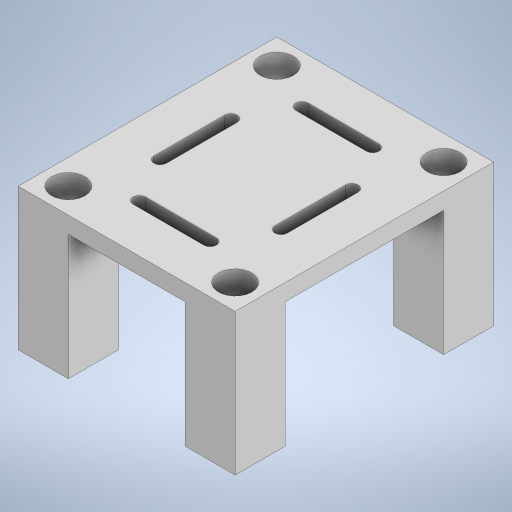
# Autodesk Inventor part: wires_keeper
Saved by Autodesk Inventor 2023 (Build 270158000, 158)
## iProperties
Created: 2023-11-26
Part Number: wires_keeper
Material: Ogólny
Document SubType Name: Modeling
Designer: janek
Density: 1 g/cm^3
Appearance: Domyślna
Author: janek
## iProperties of the stored document wires_keeper_Drukowanie 3D.ipt
Created: 2023-11-26
Part Number: wires_keeper_Drukowanie 3D
Material: Ogólny
Document SubType Name: Modeling
Designer: janek
Density: 1 g/cm^3
Appearance: Domyślna
Author: janek
Autodesk Inventor part; units mm, degrees
ref_plane "YZ Plane" through (0, 0, 0) normal (1, 0, 0) x (0, 1, 0)
ref_plane "XZ Plane" through (0, 0, 0) normal (0, 1, 0) x (-1, 0, 0)
ref_plane "XY Plane" through (0, 0, 0) normal (0, 0, 1) x (1, 0, 0)
sketch "Szkic1" plane through (0, 0, 0) normal (0, 1, 0) x (-1, 0, 0)
  line L0 (20, 25) -> (-20, 25)
  line L1 (-20, 25) -> (-20, -25)
  line L2 (-20, -25) -> (20, -25)
  line L3 (20, -25) -> (20, 25)
  line L4 (20, 25) -> (-20, -25) construction
  line L5 (-20, 25) -> (20, -25) construction
  line L6 (26, 31) -> (14, 31)
  line L7 (14, 31) -> (14, 19)
  line L8 (14, 19) -> (26, 19)
  line L9 (26, 19) -> (26, 31)
  line L10 (26, 31) -> (14, 19) construction
  line L11 (14, 31) -> (26, 19) construction
  line L12 (26, -19) -> (14, -19)
  line L13 (14, -19) -> (14, -31)
  line L14 (14, -31) -> (26, -31)
  line L15 (26, -31) -> (26, -19)
  line L16 (26, -19) -> (14, -31) construction
  line L17 (14, -19) -> (26, -31) construction
  line L18 (-14, 31) -> (-26, 31)
  line L19 (-26, 31) -> (-26, 19)
  line L20 (-26, 19) -> (-14, 19)
  line L21 (-14, 19) -> (-14, 31)
  line L22 (-14, 31) -> (-26, 19) construction
  line L23 (-26, 31) -> (-14, 19) construction
  line L24 (-14, -19) -> (-26, -19)
  line L25 (-26, -19) -> (-26, -31)
  line L26 (-26, -31) -> (-14, -31)
  line L27 (-14, -31) -> (-14, -19)
  line L28 (-14, -19) -> (-26, -31) construction
  line L29 (-26, -19) -> (-14, -31) construction
  point P0 (0, 0)
  point P1 (20, 19)
  point P2 (-14, -25)
  point P3 (-26, -25)
  point P4 (-20, -19)
  point P5 (-20, -31)
  dimension "d0" = 50
  dimension "d1" = 40
  dimension "d2" = 12
  dimension "d3" = 12
  dimension "d4" = 12
  dimension "d5" = 12
  dimension "d6" = 12
  dimension "d7" = 12
  dimension "d8" = 12
  dimension "d9" = 12
  constraints: 60 end point, 15 midpoint, 10 parallel, 5 horizontal, 5 perpendicular
  measures "d0" distance between parallel lines of L0 L2
  measures "d1" distance between parallel lines of L3 L1
  measures "d2" distance of L8.end L7.end
  measures "d3" distance from line of point (20, 19) L6
  measures "d4" distance of L14.end L13.end
  measures "d5" distance between parallel lines of L14 L12
  measures "d6" distance between parallel lines of L21 L19
  measures "d7" distance between parallel lines of L18 L20
  measures "d8" distance of point (-14, -25) point (-26, -25)
  measures "d9" distance of point (-20, -19) point (-20, -31)
extrude "Wyciągnięcie proste1" add sketch "Szkic1" along normal blind 30 contours L3 L8 L7 L0 | L0 L7 L6 L9 L8 L3 | L21 L20 L1 L0 | L0 L1 L20 L19 L18 L21 | L12 L15 L14 L13 L2 L3 | L3 L2 L13 L12 | L24 L27 L2 L1 | L1 L2 L27 L26 L25 L24
sketch "Szkic2" plane through (0, 30, 0) normal (0, 1, 0) x (1, 0, 0)
  line L0 (-26, -19) -> (-26, -31) projected
  line L1 (26, 31) -> (14, 31) projected
  line L2 (-26, -31) -> (26, -31)
  line L3 (26, -31) -> (26, 31)
  line L4 (26, 31) -> (-26, 31)
  line L5 (-26, 31) -> (-26, -31)
  point P0 (0, 0)
  constraints: 8 end point, 2 parallel, 1 horizontal, 1 perpendicular
extrude "Wyciągnięcie proste2" add sketch "Szkic2" along normal blind 4
sketch "Szkic3" plane through (0, 0, 0) normal (0, -1, 0) x (1, 0, 0)
  circle A0 centre (-20, 25) radius 2.5
  circle A1 centre (20, 25) radius 2.5
  circle A2 centre (-20, -25) radius 2.5
  circle A3 centre (20, -25) radius 2.5
  line L0 (-14, 19) -> (-26, 19) projected
  line L1 (26, 19) -> (14, 19) projected
  line L2 (-26, -19) -> (-14, -19) projected
  line L3 (14, -19) -> (26, -19) projected
  line L4 (14, -31) -> (14, -19) projected
  line L5 (-26, -31) -> (-26, -19) projected
  line L6 (-26, 19) -> (-26, 31) projected
  line L7 (14, 19) -> (14, 31) projected
  point P0 (0, 0)
  point P1 (-20, 19)
  point P2 (-20, -19)
  point P3 (-26, -25)
  dimension "d14" = 5
  dimension "d15" = 6
  dimension "d16" = 6
  dimension "d17" = 6
  dimension "d18" = 6
  dimension "d19" = 6
  dimension "d20" = 6
  dimension "d21" = 6
  dimension "d22" = 6
  dimension "d23" = 5
  dimension "d24" = 5
  dimension "d25" = 5
  constraints: 4 centre point, 3 midpoint
  measures "d14" diameter of A2
  measures "d15" distance of point (-20, 19) A0.centre
  measures "d16" distance from line of L1 A1.centre
  measures "d17" distance of A2.centre point (-20, -19)
  measures "d18" distance from line of L3 A3.centre
  measures "d19" distance from line of L4 A3.centre
  measures "d20" distance of point (-26, -25) A2.centre
  measures "d21" distance from line of L6 A0.centre
  measures "d22" distance from line of L7 A1.centre
  measures "d23" diameter of A0
  measures "d24" diameter of A1
  measures "d25" diameter of A3
extrude "Wyciągnięcie proste3" cut sketch "Szkic3" against normal blind 34
sketch "Szkic4" plane through (0, 34, 0) normal (0, 1, 0) x (1, 0, 0)
  circle A0 centre (20, 25) radius 2.5 projected
  circle A1 centre (20, 25) radius 4
  circle A2 centre (20, -25) radius 2.5 projected
  circle A3 centre (20, -25) radius 4
  circle A4 centre (-20, -25) radius 2.5 projected
  circle A5 centre (-20, -25) radius 4
  circle A6 centre (-20, 25) radius 2.5 projected
  circle A7 centre (-20, 25) radius 4
  point P0 (0, 0)
  dimension "d28" = 8
  dimension "d29" = 8
  dimension "d30" = 8
  dimension "d31" = 8
  constraints: 4 centre point, 4 coincident
  measures "d28" diameter of A3
  measures "d29" diameter of A1
  measures "d30" diameter of A7
  measures "d31" diameter of A5
extrude "Wyciągnięcie proste4" cut sketch "Szkic4" against normal blind 22
sketch "Szkic5" plane through (0, 34, 0) normal (0, 1, 0) x (1, 0, 0)
  line L0 (14.5, 8.5) -> (14.5, -8.5) construction
  line L1 (13, 8.5) -> (13, -8.5)
  line L2 (16, -8.5) -> (16, 8.5)
  arc A0 (16, 8.5) -> (13, 8.5) centre (14.5, 8.5) ccw
  arc A1 (13, -8.5) -> (16, -8.5) centre (14.5, -8.5) ccw
  line L3 (8.5, 19.5) -> (-8.5, 19.5) construction
  line L4 (8.5, 21) -> (-8.5, 21)
  line L5 (-8.5, 18) -> (8.5, 18)
  arc A2 (8.5, 18) -> (8.5, 21) centre (8.5, 19.5) ccw
  arc A3 (-8.5, 21) -> (-8.5, 18) centre (-8.5, 19.5) ccw
  line L6 (-14.5, 8.5) -> (-14.5, -8.5) construction
  line L7 (-16, 8.5) -> (-16, -8.5)
  line L8 (-13, -8.5) -> (-13, 8.5)
  arc A4 (-13, 8.5) -> (-16, 8.5) centre (-14.5, 8.5) ccw
  arc A5 (-16, -8.5) -> (-13, -8.5) centre (-14.5, -8.5) ccw
  line L9 (-8.5, -19.5) -> (8.5, -19.5) construction
  line L10 (-8.5, -21) -> (8.5, -21)
  line L11 (8.5, -18) -> (-8.5, -18)
  arc A6 (-8.5, -18) -> (-8.5, -21) centre (-8.5, -19.5) ccw
  arc A7 (8.5, -21) -> (8.5, -18) centre (8.5, -19.5) ccw
  line L12 (26, 31) -> (-26, 31) projected
  line L13 (26, -31) -> (26, 31) projected
  line L14 (-26, -31) -> (26, -31) projected
  line L15 (-26, 31) -> (-26, -31) projected
  point P0 (0, 0)
  point P1 (14.5, 0)
  point P2 (0, 19.5)
  point P3 (-14.5, 0)
  point P4 (0, -19.5)
  point P5 (-16, 0)
  point P6 (-26, 0)
  point P7 (10, 19.5)
  point P8 (-10, 19.5)
  point P9 (10, -19.5)
  point P10 (-10, -19.5)
  point P11 (14.5, -10)
  point P12 (14.5, 10)
  point P13 (-14.5, -10)
  point P14 (-14.5, 10)
  dimension "d34" = 10
  dimension "d35" = 10
  dimension "d36" = 10
  dimension "d37" = 3
  dimension "d38" = 10
  dimension "d39" = 20
  dimension "d40" = 20
  dimension "d41" = 20
  dimension "d42" = 20
  dimension "d43" = 3
  dimension "d44" = 3
  dimension "d45" = 3
  dimension "d46" = 31
  dimension "d47" = 31
  dimension "d48" = 26
  dimension "d49" = 26
  constraints: 32 end point, 24 point on circle, 16 tangent, 8 centre point, 6 midpoint, 4 parallel, 3 perpendicular, 1 vertical
  measures "d34" distance between parallel lines of L12 L4
  measures "d35" distance between parallel lines of L13 L2
  measures "d36" distance between parallel lines of L14 L10
  measures "d37" distance between parallel lines of L11 L10
  measures "d38" distance of point (-16, 0) point (-26, 0)
  measures "d39" distance of point (10, 19.5) point (-10, 19.5)
  measures "d40" distance of point (10, -19.5) point (-10, -19.5)
  measures "d41" distance of point (14.5, -10) point (14.5, 10)
  measures "d42" distance of point (-14.5, -10) point (-14.5, 10)
  measures "d43" distance between parallel lines of L5 L4
  measures "d44" distance between parallel lines of L2 L1
  measures "d45" distance between parallel lines of L8 L7
  measures "d46" distance from line of L12 point (-14.5, 0)
  measures "d47" distance from line of L12 point (14.5, 0)
  measures "d48" distance from line of L13 point (0, 19.5)
  measures "d49" distance from line of L13 point (0, -19.5)
extrude "Wyciągnięcie proste5" cut sketch "Szkic5" against normal blind 22 contours A0 L2 A1 L1 | A2 L5 A3 L4 | A4 L8 A5 L7 | A6 L11 A7 L10
